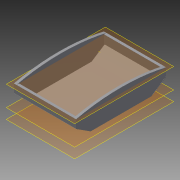
# Autodesk Inventor part: Basic Frame
Saved by Autodesk Inventor 2015 (Build 190159000, 159)
## iProperties
Created: 2016-01-18
Part Number: Basic Frame
Material: Generic
Document SubType Name: Modeling
Designer: sethbattis
Density: 1 g/cm^3
Appearance: Default
Author: sethbattis
Autodesk Inventor part; units mm, degrees
ref_plane "YZ Plane" through (0, 0, 0) normal (1, 0, 0) x (0, 1, 0)
ref_plane "XY Plane" through (0, 0, 0) normal (0, 0, 1) x (1, 0, 0)
sketch "Sketch1" plane through (0, 0, 0) normal (0, 1, 0) x (-1, 0, 0)
  line L0 (311.15, 450.85) -> (-311.15, 450.85)
  line L1 (-311.15, 450.85) -> (-311.15, -450.85)
  line L2 (-311.15, -450.85) -> (311.15, -450.85)
  line L3 (311.15, -450.85) -> (311.15, 450.85)
  line L4 (0, -631.19) -> (0, 631.19) projected
  line L5 (435.61, 0) -> (-435.61, 0) projected
  line L6 (285.75, 425.45) -> (-285.75, 425.45)
  line L7 (-285.75, 425.45) -> (-285.75, -425.45)
  line L8 (-285.75, -425.45) -> (285.75, -425.45)
  line L9 (285.75, -425.45) -> (285.75, 425.45)
  line L10 (311.15, 0) -> (285.75, 0) construction
  line L11 (0, 425.45) -> (0, 450.85) construction
  line L12 (-285.75, 0) -> (-311.15, 0) construction
  line L13 (0, -425.45) -> (0, -450.85) construction
  point P0 (0, 0)
  dimension "d0" = 622.3
  dimension "d1" = 901.7
  dimension "d2" = 311.15
  dimension "d3" = 450.85
  dimension "d4" = 25.4
  constraints: 24 end point, 8 midpoint, 8 point on line, 4 parallel, 3 equal length, 2 horizontal, 2 perpendicular
  measures "d0" distance of L2.end L1.end
  measures "d1" distance of L1.end L0.end
  measures "d2" distance between parallel lines of L3 L4
  measures "d3" distance between parallel lines of L2 L5
  measures "d4" distance between parallel lines of L9 L3
extrude "Extrusion1" add sketch "Sketch1" along normal blind 84.1375 contours L3 L5 L9 L6 L4 L0 | L4 L6 L7 L5 L1 L0 | L3 L2 L4 L8 L9 L5 | L5 L7 L8 L4 L2 L1
sketch "Sketch2" plane through (311.15, 0, 450.85) normal (1, 0, 0) x (0, 0, -1)
  arc A0 (901.7, 84.1375) -> (0, 84.1375) centre (450.85, -1891.1094) ccw
  line L0 (-140.1666, 134.9375) -> (1288.9665, 134.9375) construction
  line L1 (-140.1666, -220.6625) -> (1288.9665, -220.6625) construction
  line L2 (0, 84.1375) -> (901.7, 84.1375) projected
  line L3 (-140.1666, -93.6625) -> (1288.9665, -93.6625) construction
  line L4 (450.85, 187.6829) -> (450.85, -340.5208) construction
  line L5 (146.05, 172.3928) -> (146.05, -340.5208) construction
  line L6 (755.65, 187.6829) -> (755.65, -330.7907) construction
  line L7 (-140.1666, 134.9375) -> (-140.1666, -220.6625) construction
  line L8 (0, 0) -> (901.7, 0) projected
  line L9 (0, 0) -> (146.05, -93.6625)
  line L10 (755.65, -93.6625) -> (901.7, 0)
  line L11 (146.05, -93.6625) -> (755.65, -93.6625)
  line L12 (0, 84.1375) -> (0, 0)
  line L13 (0, 0) -> (0, 84.1375) projected
  line L14 (901.7, 84.1375) -> (901.7, 0)
  point P0 (450.85, 0)
  point P1 (450.85, 0)
  dimension "d8" = 355.6
  dimension "d9" = 50.8
  dimension "d10" = 127
  dimension "d11" = 304.8
  dimension "d12" = 304.8
  constraints: 24 end point, 6 point on line, 4 vertical, 3 horizontal, 2 collinear, 2 parallel, 2 point on circle, 1 centre point, 1 midpoint, 1 perpendicular, 1 tangent
  measures "d8" distance between parallel lines of L1 L0
  measures "d9" distance between parallel lines of L0 L2
  measures "d10" distance between parallel lines of L1 L3
  measures "d11" distance between parallel lines of L4 L5
  measures "d12" distance between parallel lines of L6 L4
extrude "Extrusion2" add sketch "Sketch2" against normal blind 25.4
mirror "Mirror3" about plane through (0, 0, 0) normal (1, 0, 0) of "Extrusion2"
ref_plane "Ground Plane" through (0, -220.9292, 0) normal (0, 1, 0) x (-1, 0, 0)
ref_plane "Work Plane3" through (-285.75, -46.8313, -377.825) normal (0, -0.5398324, 0.8417725) x (1, 0, 0)
sketch "Sketch4" plane through (311.15, -1891.1094, 0) normal (1, 0, 0) x (0, 0, -1)
  line L0 (-450.85, 1891.1094) -> (-304.8, 1797.4469)
  line L1 (-450.85, 1891.1094) -> (-304.8, 1797.4469) projected
  line L2 (-304.8, 1797.4469) -> (304.8, 1797.4469)
  line L3 (304.8, 1797.4469) -> (450.85, 1891.1094)
  line L4 (450.85, 1891.1094) -> (304.8, 1797.4469) projected
  line L5 (450.85, 1891.1094) -> (449.136, 1893.782)
  line L6 (425.45, 1891.1094) -> (425.45, 1975.2469) projected
  line L7 (449.136, 1893.782) -> (303.8694, 1800.6219)
  line L8 (303.8694, 1800.6219) -> (-306.8101, 1800.6219)
  line L9 (-306.8101, 1800.6219) -> (-449.993, 1892.4457)
  line L10 (-450.85, 1891.1094) -> (-449.136, 1893.782)
  point P0 (0, 1891.1094)
  dimension "d18" = 3.175
  dimension "d20" = 3.175
  dimension "d21" = 3.175
  constraints: 16 end point, 2 collinear, 2 parallel, 2 perpendicular, 1 horizontal, 1 midpoint
  measures "d18" distance of L3.end L5.end
  measures "d20" distance of L0.start L10.end
  measures "d21" distance between parallel lines of L2 L8
extrude "Extrusion5" add sketch "Sketch4" against normal blind 622.3 separate body
ref_plane "Lower Bumper Plane" through (0, -119.3292, 0) normal (0, 1, 0) x (-1, 0, 0)
ref_plane "Upper Bumper Plane" through (0, 83.8708, 0) normal (0, 1, 0) x (-1, 0, 0)
equation "\"d2\" = 0.5 * d0"
equation "\"d3\" = 0.5 * d1"
body "Solid1"
body "Solid2"
